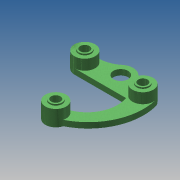
# Autodesk Inventor part: Linearwagen_MauroW_inside
Saved by Autodesk Inventor 2015 SP1 (Build 190203100, 203)
## iProperties
Created: 2015-02-25
Part Number: Linearwagen_MauroW_inside
Material: Generisch
Document SubType Name: Modeling
Designer: Marc
Density: 1 g/cm^3
Appearance: Gehont - dunkelgrau(2)
Author: Marc
Autodesk Inventor part; units mm, degrees
ref_plane "YZ Plane" through (0, 0, 0) normal (1, 0, 0) x (0, 1, 0)
ref_plane "XZ Plane" through (0, 0, 0) normal (0, 1, 0) x (-1, 0, 0)
ref_plane "XY Plane" through (0, 0, 0) normal (0, 0, 1) x (1, 0, 0)
sketch "Skizze1" plane through (0, 0, 0) normal (0, 0, 1) x (1, 0, 0)
  line L0 (-50.1686, 0) -> (50.7617, 0) projected
  line L1 (0, -73.5762) -> (0, 44.2069) projected
  circle A0 centre (-21, 0) radius 3.35
  circle A1 centre (-21, 0) radius 14.75 construction
  circle A2 centre (21, 0) radius 3.35
  circle A3 centre (21, 0) radius 14.75 construction
  circle A4 centre (0, -42) radius 3.35
  circle A5 centre (0, -42) radius 14.75 construction
  circle A6 centre (0, 5) radius 5.3
  circle A7 centre (0, 5) radius 9
  circle A8 centre (-21, 0) radius 7.5
  circle A9 centre (21, 0) radius 7.5
  arc A10 (-20.3023, 7.4675) -> (-5.7233, 11.9458) centre (-18.4418, 27.3808) ccw
  arc A11 (5.7233, 11.9458) -> (20.3023, 7.4675) centre (18.4418, 27.3808) ccw
  line L2 (-21, -7.5) -> (21, -7.5)
  circle A12 centre (0, -42) radius 7.5
  arc A13 (3.6768, -35.4631) -> (14.5419, -3.8136) centre (-4.4018, -15) ccw
  arc A14 (7.272, -43.8351) -> (28.2692, 1.8462) centre (-10.5, -8) ccw
  point P0 (0, 0)
  point P1 (28.1068, -2.3967)
  point P2 (19.4082, -7.3291)
  point P3 (-19.4082, -7.3291)
  point P4 (13.6211, 1.3423)
  point P5 (2.9103, -48.9123)
  point P6 (28.4986, 0.1465)
  point P7 (-0.3947, -34.5104)
  point P8 (13.9951, -2.6799)
  dimension "d16" = 15
  dimension "d0" = 6.7
  dimension "d3" = 29.5
  dimension "d4" = 21
  dimension "d5" = 6.7
  dimension "d6" = 42
  dimension "d7" = 29.5
  dimension "d12" = 10.6
  dimension "d13" = 18
  dimension "d14" = 5
  dimension "d15" = 15
  dimension "d19" = 20
  dimension "d20" = 20
  dimension "d47" = 15
  dimension "d51" = 22
  dimension "d52" = 40
  dimension "d53" = 27
  dimension "d54" = 34
  constraints: 17 point on circle, 14 centre point, 7 coincident, 3 point on line, 3 tangent, 2 end point, 2 horizontal, 2 symmetric about line, 16 other
  measures "d0" diameter of A0
  measures "d3" diameter of A1
  measures "d4" distance of point (0, 0) A0.centre
  measures "d5" diameter of A4
  measures "d6" distance of point (0, 0) A4.centre
  measures "d7" diameter of A5
  measures "d12" diameter of A6
  measures "d13" diameter of A7
  measures "d14" distance from line of L0 A6.centre
  measures "d15" diameter of A8
  measures "d19" radius of A10
  measures "d20" radius of A11
  measures "d47" diameter of A12
  measures "d51" radius of A13
  measures "d52" radius of A14
  measures "d53" vertical distance of A12.centre A13.centre
  measures "d54" vertical distance of A12.centre A14.centre
extrude "Extrusion1" add sketch "Skizze1" against normal blind 4 contours A0 L0 A8 | L0 A8 A0 | A8 A10 A7 L0 | L0 A7 L1 L2 A8 | A7 L1 A6 L0 | L0 A6 L1 A7 | A7 L0 A9 A13 L2 L1 | L1 A6 L0 A7 | L1 A7 L0 A6 | A7 A11 A9 L0 | A12 L1 A4 | L1 A4 A12 | A13 A9 L2 | L2 A9 L0 A14 A12 A13 | A9 L0 A2 | L0 A2 A9 | A9 A14 L0
sketch "Skizze4" plane through (0, 0, -4) normal (0, 0, -1) x (-1, 0, 0)
  circle A0 centre (-21, 0) radius 3.35 projected
  circle A1 centre (0, 5) radius 5.3 projected
  circle A2 centre (21, 0) radius 3.35 projected
  line L0 (-16.2803, -7.5) -> (21, -7.5) projected
  arc A3 (21, -7.5) -> (20.3023, 7.4675) centre (21, 0) ccw projected
  arc A4 (5.7233, 11.9458) -> (20.3023, 7.4675) centre (18.4418, 27.3808) ccw projected
  arc A5 (5.7233, 11.9458) -> (-5.7233, 11.9458) centre (0, 5) ccw projected
  arc A6 (-20.3023, 7.4675) -> (-5.7233, 11.9458) centre (-18.4418, 27.3808) ccw projected
  arc A7 (-20.3023, 7.4675) -> (-28.2692, 1.8462) centre (-21, 0) ccw projected
  circle A8 centre (-21, 0) radius 7.5
  circle A9 centre (21, 0) radius 7.5
  arc A10 (-7.272, -43.8351) -> (-3.6768, -35.4631) centre (0, -42) ccw projected
  arc A11 (-28.2692, 1.8462) -> (-7.272, -43.8351) centre (10.5, -8) ccw projected
  arc A12 (-16.2803, -7.5) -> (-3.6768, -35.4631) centre (4.4018, -15) ccw projected
  point P0 (0, 0)
  dimension "d34" = 15
  dimension "d35" = 15
  constraints: 2 centre point, 2 coincident
  measures "d34" diameter of A8
  measures "d35" diameter of A9
extrude "Extrusion4" add sketch "Skizze4" along normal blind 7.5 contours A9 A3 | A7 A8
sketch "Skizze5" plane through (21, 0, -11.5) normal (0, 0, -1) x (-1, 0, 0)
  circle A0 centre (0, 0) radius 3.35 projected
  circle A1 centre (0, 0) radius 7.5 projected
  circle A2 centre (42, 0) radius 3.35 projected
  circle A3 centre (42, 0) radius 7.5 projected
  circle A4 centre (0, 0) radius 4.5
  circle A5 centre (42, 0) radius 3.4 projected
  circle A6 centre (42, 0) radius 4.5
  point P0 (21, 0)
  dimension "d38" = 9
  dimension "d39" = 9
  constraints: 2 centre point, 2 coincident
  measures "d38" diameter of A4
  measures "d39" diameter of A6
extrude "Extrusion5" add sketch "Skizze5" along normal blind 1 contours A4 | A5 | A6
sketch "Skizze8" plane through (0, 0, -4) normal (0, 0, -1) x (-1, 0, 0)
  circle A0 centre (0, -42) radius 3.35 projected
  circle A1 centre (0, 5) radius 5.3 projected
  arc A2 (-28.2692, 1.8462) -> (-20.3023, 7.4675) centre (-21, 0) ccw projected
  arc A3 (-28.2692, 1.8462) -> (-7.272, -43.8351) centre (10.5, -8) ccw projected
  arc A4 (-7.272, -43.8351) -> (-3.6768, -35.4631) centre (0, -42) ccw projected
  arc A5 (-16.2803, -7.5) -> (-3.6768, -35.4631) centre (4.4018, -15) ccw projected
  line L0 (-16.2803, -7.5) -> (21, -7.5) projected
  arc A6 (20.3023, 7.4675) -> (21, -7.5) centre (21, 0) ccw projected
  arc A7 (5.7233, 11.9458) -> (20.3023, 7.4675) centre (18.4418, 27.3808) ccw projected
  arc A8 (5.7233, 11.9458) -> (-5.7233, 11.9458) centre (0, 5) ccw projected
  arc A9 (-20.3023, 7.4675) -> (-5.7233, 11.9458) centre (-18.4418, 27.3808) ccw projected
  circle A10 centre (0, -42) radius 7.5
  point P0 (0, 0)
  dimension "d55" = 15
  constraints: 1 centre point, 1 coincident
  measures "d55" diameter of A10
extrude "Extrusion7" add sketch "Skizze8" along normal blind 7.5 contours A10 A4
sketch "Skizze9" plane through (0, -42, -11.5) normal (0, 0, -1) x (-1, 0, 0)
  circle A0 centre (0, 0) radius 3.35 projected
  circle A1 centre (0, 0) radius 7.5 projected
  circle A2 centre (0, 0) radius 4.5
  point P0 (0, 42)
  dimension "d58" = 9
  constraints: 1 centre point, 1 coincident
  measures "d58" diameter of A2
extrude "Extrusion8" add sketch "Skizze9" along normal blind 1 contours A2
mirror "Spiegeln1" about plane through (0, 0, 0) normal (0, 0, 1) of "Extrusion1", "Extrusion4", "Extrusion5", "Extrusion7", "Extrusion8"
sketch "Skizze19" plane through (0, 0, 0) normal (0, 0, 1) x (1, 0, 0)
  line L0 (-37.3748, -55.7465) -> (60.3793, -55.7465)
  line L1 (60.3793, -55.7465) -> (60.3793, 24.5119)
  line L2 (60.3793, 24.5119) -> (-37.3748, 24.5119)
  line L3 (-37.3748, 24.5119) -> (-37.3748, -55.7465)
  point P0 (0, 0)
  constraints: 8 end point, 2 parallel, 1 horizontal, 1 perpendicular
extrude "Extrusion17" cut sketch "Skizze19" against normal blind 13
equation "\"d5\" = d0"
equation "\"d7\" = d3"
equation "\"d20\" = d19"
